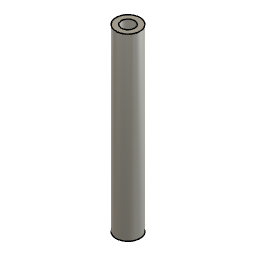
BC linaer drive motor spacer v3 (Autodesk Fusion 360 design; units mm, degrees)
Autodesk Fusion 360 part; units mm, degrees
cylinder "CylinderPrimitive1" add diameter 10 height 75 placed x (1, 0, 0) y (0, 0, -1) z (0, 1, 0) at (0, 0, 0)
hole "Hole1" at (0, 0, 0) direction (0, 1, 0) diameter 5.5 end through all
